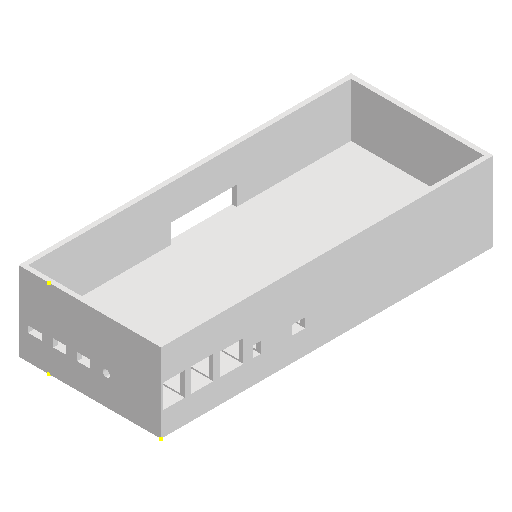
# Autodesk Inventor part: BOX_SAMPAH
Saved by Autodesk Inventor 2026.2 (Build 302298000, 298)
## iProperties
Created: 2026-01-29
Part Number: BOX_SAMPAH
Material: Generic
Document SubType Name: Modeling
Designer: defaultuser0
Density: 1 g/cm^3
Appearance: Default
Author: defaultuser0
Autodesk Inventor part; units mm, degrees
ref_plane "YZ Plane" through (0, 0, 0) normal (1, 0, 0) x (0, 1, 0)
ref_plane "XZ Plane" through (0, 0, 0) normal (0, 1, 0) x (-1, 0, 0)
ref_plane "XY Plane" through (0, 0, 0) normal (0, 0, 1) x (1, 0, 0)
sketch "Sketch1" plane through (0, 0, 0) normal (0, 0, 1) x (1, 0, 0)
  point P0 (0, 0)
sketch "Sketch2" plane through (0, 0, 0) normal (0, 0, 1) x (1, 0, 0)
  line L0 (20.0728, 0) -> (-15.1545, 0)
  line L1 (-19.19, 0) -> (-19.19, 50)
  line L2 (-19.19, 50) -> (70.81, 50)
  line L3 (70.81, 50) -> (70.81, 0)
  line L4 (70.81, 0) -> (-19.19, 0)
  line L5 (-19.19, 0) -> (-13.19, 0)
  line L6 (-13.19, 0) -> (-13.19, 15)
  point P0 (0, 0)
  dimension "d0" = 50
  dimension "d1" = 90
  dimension "d2" = 15
  dimension "d5" = 6
  constraints: 14 end point, 2 parallel, 2 perpendicular, 1 point on line, 1 vertical
  measures "d0" distance of L1.start L1.end
  measures "d1" distance of L1.end L2.end
  measures "d2" distance of L5.end L6.end
  measures "d5" distance between parallel lines of L6 L1
sketch "Sketch3" plane through (0, 0, 0) normal (0, 0, 1) x (1, 0, 0)
  line L0 (-13.1902, 15.9972) -> (-4.1902, 15.9972)
  line L1 (-4.1902, 15.9972) -> (-4.1902, 19.9972)
  line L2 (-4.1902, 19.9972) -> (-13.1902, 19.9972)
  line L3 (-13.1902, 19.9972) -> (-13.1902, 15.9972)
  line L4 (2.8098, 15.9972) -> (2.8098, 20.9972)
  line L5 (2.8098, 20.9972) -> (10.8098, 20.9972)
  line L6 (10.8098, 20.9972) -> (10.8098, 15.9972)
  line L7 (10.8098, 15.9972) -> (2.8098, 15.9972)
  line L8 (2.8098, 15.9972) -> (2.8098, 20.9972)
  line L9 (2.8098, 20.9972) -> (10.8098, 20.9972)
  line L10 (10.8098, 20.9972) -> (10.8098, 15.9972)
  line L11 (10.8098, 15.9972) -> (2.8098, 15.9972)
  line L12 (17.8096, 15.9972) -> (17.8096, 20.9972)
  line L13 (17.8096, 20.9972) -> (25.8096, 20.9972)
  line L14 (25.8096, 20.9972) -> (25.8096, 15.9972)
  line L15 (25.8096, 15.9972) -> (17.8096, 15.9972)
  line L16 (17.8096, 15.9972) -> (17.8096, 20.9972)
  line L17 (17.8096, 20.9972) -> (25.8096, 20.9972)
  line L18 (25.8096, 20.9972) -> (25.8096, 15.9972)
  line L19 (25.8096, 15.9972) -> (17.8096, 15.9972)
  circle A0 centre (36.289, 18.4972) radius 2.2825
  point P0 (0, 0)
  dimension "d7" = 9
  dimension "d8" = 4
  dimension "d9" = 9
  dimension "d11" = 5
  dimension "d12" = 8
  dimension "d13" = 5
  dimension "d14" = 8
  dimension "d16" = 7
  dimension "d18" = 5
  dimension "d19" = 8
  dimension "d20" = 5
  dimension "d21" = 8
  dimension "d22" = 5
  dimension "d23" = 8
  dimension "d24" = 5
  dimension "d25" = 8
  dimension "d27" = 5
  dimension "d28" = 8
  dimension "d29" = 5
  dimension "d30" = 8
  constraints: 40 end point, 5 perpendicular, 1 centre point
  measures "d7" distance of L0.start L0.end
  measures "d8" distance of L0.end L1.end
  measures "d9" distance of L1.end L2.end
  measures "d11" distance of L4.start L4.end
  measures "d12" distance of L4.end L5.end
  measures "d13" distance of L5.end L6.end
  measures "d14" distance of L6.end L4.start
  measures "d16" distance of L0.end L4.start
  measures "d18" distance of L8.start L8.end
  measures "d19" distance of L8.end L9.end
  measures "d20" distance of L9.end L10.end
  measures "d21" distance of L10.end L8.start
  measures "d22" distance of L12.start L12.end
  measures "d23" distance of L12.end L13.end
  measures "d24" distance of L13.end L14.end
  measures "d25" distance of L14.end L12.start
  measures "d27" distance of L16.start L16.end
  measures "d28" distance of L16.end L17.end
  measures "d29" distance of L17.end L19.start
  measures "d30" distance of L19.start L16.start
sketch "Sketch4" plane through (0, 0, 0) normal (1, 0, 0) x (0, 1, 0)
  point P0 (0, 0)
sketch "Sketch5" plane through (0, 0, 0) normal (1, 0, 0) x (0, 1, 0)
  point P0 (0, 0)
sketch "Sketch6" plane through (0, 0, 0) normal (1, 0, 0) x (0, 1, 0)
  point P0 (0, 0)
extrude "Extrusion2" add sketch "Sketch2" against normal blind 210
sketch "Sketch7" plane through (70.81, 0, 0) normal (1, 0, 0) x (0, 0, -1)
  point P0 (0, 0)
sketch "Sketch8" plane through (-19.19, 50, 0) normal (0, 1, 0) x (1, 0, 0)
  point P0 (19.19, 0)
sketch "Sketch9" plane through (-19.19, 50, 0) normal (0, 1, 0) x (1, 0, 0)
  line L0 (0, 210) -> (90, 210) projected
  line L1 (0, 210) -> (3, 210)
  line L2 (3, 210) -> (0, 210)
  line L3 (90, 210) -> (87, 210)
  line L4 (90, 0) -> (0, 0) projected
  line L5 (90, 0) -> (90, 210) projected
  line L6 (90, 3) -> (90, 0)
  line L7 (0, 0) -> (0, 3)
  line L8 (0, 0) -> (0, 210) projected
  line L9 (3, 207) -> (87, 207)
  line L10 (87, 207) -> (87, 3)
  line L11 (87, 3) -> (3, 3)
  line L12 (3, 3) -> (3, 207)
  point P0 (19.19, 0)
  dimension "d39" = 3
  dimension "d40" = 3
  constraints: 18 end point, 4 point on line, 2 collinear, 2 parallel, 1 perpendicular
  measures "d39" distance of L0.start L1.end
  measures "d40" distance of L1.end L0.start
extrude "Extrusion3" cut sketch "Sketch9" against normal blind 34.03 contours L9 L10 L11 L12
extrude "Extrusion4" cut sketch "Sketch3" against normal blind 33.25
sketch "Sketch10" plane through (0, 0, 0) normal (0, 0, 1) x (1, 0, 0)
  point P0 (0, 0)
sketch "Sketch11" plane through (0, 0, 0) normal (0, 0, 1) x (1, 0, 0)
  point P0 (0, 0)
sketch "Sketch12" plane through (67.81, 50, -3) normal (0, 0, -1) x (-1, 0, 0)
  point P0 (67.81, -50)
sketch "Sketch13" plane through (67.81, 50, -3) normal (0, 0, -1) x (-1, 0, 0)
  point P0 (67.81, -50)
sketch "Sketch14" plane through (0, 0, 0) normal (0, 0, 1) x (1, 0, 0)
  point P0 (0, 0)
sketch "Sketch15" plane through (70.81, 0, 0) normal (1, 0, 0) x (0, 0, -1)
  line L0 (0, 0) -> (0, 15)
  line L1 (0, 0) -> (0, 50) projected
  line L2 (0, 15) -> (1, 15)
  line L3 (1, 15) -> (15, 15)
  line L4 (15, 15) -> (15, 30)
  line L5 (15, 30) -> (1, 30)
  line L6 (1, 30) -> (1, 15)
  line L7 (15, 15) -> (19, 15)
  line L8 (19, 15) -> (33, 15)
  line L9 (33, 15) -> (33, 30)
  line L10 (33, 30) -> (19, 30)
  line L11 (19, 30) -> (19, 15)
  line L12 (33, 15) -> (37, 15)
  line L13 (37, 15) -> (52, 15)
  line L14 (52, 15) -> (52, 29)
  line L15 (52, 29) -> (37, 29)
  line L16 (37, 29) -> (37, 15)
  line L17 (52, 15) -> (58, 15)
  line L18 (58, 15) -> (63, 15)
  line L19 (63, 15) -> (63, 22)
  line L20 (63, 22) -> (58, 22)
  line L21 (58, 22) -> (58, 15)
  line L22 (63, 15) -> (83, 15)
  line L23 (83, 15) -> (91, 15)
  line L24 (91, 15) -> (91, 21)
  line L25 (91, 21) -> (83, 21)
  line L26 (83, 21) -> (83, 15)
  dimension "d53" = 15
  dimension "d54" = 1
  dimension "d55" = 14
  dimension "d56" = 15
  dimension "d57" = 4
  dimension "d58" = 14
  dimension "d59" = 15
  dimension "d60" = 4
  dimension "d61" = 15
  dimension "d62" = 14
  dimension "d63" = 6
  dimension "d64" = 5
  dimension "d65" = 7
  dimension "d66" = 20
  dimension "d67" = 8
  dimension "d68" = 6
  constraints: 52 end point, 10 parallel, 9 horizontal, 6 perpendicular, 1 point on line
  measures "d53" distance of L0.start L0.end
  measures "d54" distance of L0.end L2.end
  measures "d55" distance of L5.end L4.end
  measures "d56" distance of L3.end L4.end
  measures "d57" distance of L3.end L7.end
  measures "d58" distance of L10.end L9.end
  measures "d59" distance of L8.end L9.end
  measures "d60" distance of L8.end L12.end
  measures "d61" distance of L15.end L14.end
  measures "d62" distance of L13.end L14.end
  measures "d63" distance of L13.end L17.end
  measures "d64" distance of L20.end L19.end
  measures "d65" distance of L18.end L19.end
  measures "d66" distance of L18.end L22.end
  measures "d67" distance of L25.end L24.end
  measures "d68" distance of L23.end L24.end
extrude "Extrusion5" cut sketch "Sketch15" against normal blind 15.5
sketch "Sketch16" plane through (-19.19, 0, 0) normal (-1, 0, 0) x (0, 0, 1)
  line L0 (-3, 15.97) -> (-207, 15.97) projected
  line L1 (-134.7114, 15.97) -> (-93.0359, 15.97)
  line L2 (-93.0359, 15.97) -> (-93.0359, 28.1023)
  line L3 (-93.0359, 28.1023) -> (-134.7114, 28.1023)
  line L4 (-134.7114, 28.1023) -> (-134.7114, 15.97)
  point P0 (0, 0)
  constraints: 8 end point, 2 parallel, 1 horizontal, 1 perpendicular, 1 point on line
extrude "Extrusion6" cut sketch "Sketch16" against normal blind 14.25
body "Solid2"
